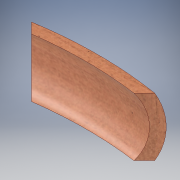
# Autodesk Inventor part: dou_short_round
Saved by Autodesk Inventor 2019 (Build 230136000, 136)
## iProperties
Created: 2019-11-15
Part Number: dou_short_round
Material: Красное дерево
Document SubType Name: Modeling
Designer: stepa
Density: 0.512 g/cm^3
Appearance: Красное дерево — натуральный — полированный
Mass: 93.7928 g
Surface Area: 359.504 cm^2
Volume: 183.189 cm^3
Author: stepa
Autodesk Inventor part; units mm, degrees
ref_plane "YZ Plane" through (0, 0, 0) normal (1, 0, 0) x (0, 1, 0)
ref_plane "XZ Plane" through (0, 0, 0) normal (0, 1, 0) x (-1, 0, 0)
ref_plane "XY Plane" through (0, 0, 0) normal (0, 0, 1) x (1, 0, 0)
sketch "Эскиз1" plane through (0, 0, 0) normal (0, 1, 0) x (-1, 0, 0)
  line L0 (0, 0) -> (-200, 0)
  line L1 (-200, 0) -> (-200, -30)
  line L2 (-200, -30) -> (0, -30)
  line L3 (0, -30) -> (0, 0)
  dimension "d0" = 200
  dimension "d1" = 30
  constraints: 8 end point, 2 parallel, 1 horizontal, 1 perpendicular
  measures "d0" distance of L2.end L1.end
  measures "d1" distance of L1.end L0.end
extrude "Выдавливание1" add sketch "Эскиз1" along normal blind 80
chamfer "Фаска1" distance 30 angle 45 2 edges at (0, 40, 0) (200, 40, 0)
sketch "Эскиз3" plane through (0, 80, 0) normal (0, 1, 0) x (1, 0, 0)
  line L0 (200, 30) -> (170, 0) projected
  line L1 (200, 30) -> (0, 30) projected
  line L2 (30, 0) -> (0, 30) projected
  line L3 (30, 0) -> (170, 0) projected
  line L4 (30, 0) -> (0, 30) projected
  line L5 (15, 15) -> (7.9289, 22.0711)
  arc A0 (192.0711, 22.0711) -> (7.9289, 22.0711) centre (100, -508.5309) ccw
  line L6 (200, 30) -> (0, 30) projected
  line L7 (30, 0) -> (170, 0) projected
  arc A1 (170, 0) -> (30, 0) centre (100, -508.5309) ccw
  point P0 (0, 0)
  point P1 (100, 0)
  point P2 (100, 0)
  dimension "d11" = 10
  constraints: 4 point on circle, 3 midpoint, 2 centre point, 2 end point, 2 point on line, 2 vertical alignment, 1 concentric, 1 tangent
  measures "d11" distance of L5.start L5.end
extrude "Выдавливание3" cut sketch "Эскиз3" against normal through all contours L0 A0 L1 | A0 L2 L1 | L3 A1
sketch "Эскиз4" plane through (192.0711, 0, -22.0711) normal (0.7071068, 0, 0.7071068) x (0.7071068, 0, -0.7071068)
  line L0 (0, 0) -> (0, 80) projected
  line L1 (0, 80) -> (-31.2132, 80) projected
  line L2 (-31.2132, 80) -> (-31.2132, 0) projected
  line L3 (-31.2132, 0) -> (0, 0) projected
  line L4 (0, 80) -> (-130.2082, 80) projected
  arc A0 (-11.2132, 0) -> (-11.2132, 80) centre (-76.9511, 40) ccw
  arc A1 (-31.2132, 0) -> (-31.2132, 80) centre (-76.9511, 40) ccw
  line L5 (-31.2132, 0) -> (0, 0) projected
  line L6 (0, 0) -> (0, 80) projected
  line L7 (-31.2132, 80) -> (-11.2132, 80)
  line L8 (-31.2132, 0) -> (-11.2132, 0)
  point P0 (-151.4214, 0)
  point P1 (-31.2132, 40)
  dimension "d14" = 20
  constraints: 4 end point, 4 point on circle, 2 centre point, 2 collinear, 2 point on line, 1 coincident, 1 concentric, 1 horizontal alignment, 1 midpoint, 1 tangent
  measures "d14" distance of L7.end L1.end
sketch3d "3D эскиз1"
  arc A0 (192.0711, 80, -22.0711) -> (7.9289, 80, -22.0711) centre (100, 80, 508.5309) ccw
sweep "Сдвиг1" cut profiles "Эскиз4" path "3D эскиз1" contours L3 A0 L0 | A0 L1 L0 | L2 A1
